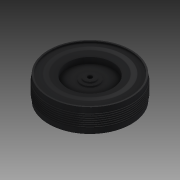
# Autodesk Inventor part: wheel
Saved by Autodesk Inventor 2016 (Build 200138000, 138)
## iProperties
Created: 2014-07-17
Part Number: wheel
Material: Rubber
Document SubType Name: Modeling
Designer: Sebastian
Density: 0.93 g/cm^3
Appearance: Rubber - Black - Version 1.1
Mass: 14.4861 g
Surface Area: 122.357 cm^2
Volume: 15.5764 cm^3
Author: Sebastian
Autodesk Inventor part; units mm, degrees
ref_plane "YZ Plane" through (0, 0, 0) normal (1, 0, 0) x (0, 1, 0)
ref_plane "XZ Plane" through (0, 0, 0) normal (0, 1, 0) x (-1, 0, 0)
ref_plane "XY Plane" through (0, 0, 0) normal (0, 0, 1) x (1, 0, 0)
sketch "Sketch1" plane through (0, 0, 0) normal (0, 1, 0) x (-1, 0, 0)
  line L0 (0, -15.5) -> (3, -15.5)
  line L1 (3, -15.5) -> (3, -3)
  line L2 (3, -3) -> (10, -3)
  line L3 (10, -3) -> (10, -8)
  line L4 (10, -8) -> (23, -8)
  line L5 (23, -8) -> (23, -19)
  line L6 (23, -19) -> (26, -19)
  line L7 (12.5, -1) -> (12.5, -5)
  line L8 (26, -19) -> (26, -5)
  line L9 (27.5, -32.1493) -> (27.5, 12.13)
  line L10 (26, -5) -> (26, -2)
  line L11 (26, -2) -> (23.5, -2)
  line L12 (23.5, -2) -> (23.5, -3)
  line L13 (23.5, -3) -> (21.5, -3)
  line L14 (21.5, -3) -> (21.5, -4)
  arc A0 (21.5, -4) -> (12.5, -5) centre (20.6098, -36.988) ccw
  line L15 (0, -15.5) -> (0, -11.75)
  line L16 (0, 0) -> (0, -3.75)
  line L17 (0, -11.75) -> (-0.5, -11.75)
  line L18 (-0.5, -11.75) -> (-0.5, -11.25)
  line L19 (-0.5, -11.25) -> (0, -11.25)
  line L20 (0, -11.25) -> (0, -10.5)
  line L21 (0, -10.5) -> (-0.5, -10.5)
  line L22 (-0.5, -10.5) -> (-0.5, -10)
  line L23 (-0.5, -10) -> (0, -10)
  line L24 (0, -10) -> (0, -9.25)
  line L25 (0, -9.25) -> (-0.5, -9.25)
  line L26 (-0.5, -9.25) -> (-0.5, -8.75)
  line L27 (-0.5, -8.75) -> (0, -8.75)
  line L28 (0, -8.75) -> (0, -8)
  line L29 (0, -8) -> (-0.5, -8)
  line L30 (-0.5, -8) -> (-0.5, -7.5)
  line L31 (-0.5, -7.5) -> (0, -7.5)
  line L32 (0, -7.5) -> (0, -6.75)
  line L33 (0, -6.75) -> (-0.5, -6.75)
  line L34 (-0.5, -6.75) -> (-0.5, -6.25)
  line L35 (-0.5, -6.25) -> (0, -6.25)
  line L36 (0, -6.25) -> (0, -5.5)
  line L37 (0, -5.5) -> (-0.5, -5.5)
  line L38 (-0.5, -5.5) -> (-0.5, -5)
  line L39 (-0.5, -5) -> (0, -5)
  line L40 (0, -5) -> (0, -4.25)
  line L41 (0, -4.25) -> (-0.5, -4.25)
  line L42 (-0.5, -4.25) -> (-0.5, -3.75)
  line L43 (-0.5, -3.75) -> (0, -3.75)
  line L44 (0, 0) -> (1, 0)
  line L45 (1, 0) -> (1, -1)
  arc A1 (12.5, -1) -> (1, -1) centre (6.75, -17.0302) ccw
  dimension "d0" = 15.5
  dimension "d1" = 3
  dimension "d2" = 12.5
  dimension "d3" = 7
  dimension "d4" = 5
  dimension "d5" = 13
  dimension "d6" = 11
  dimension "d8" = 3
  dimension "d10" = 4
  dimension "d11" = 13.5
  dimension "d12" = 26
  dimension "d16" = 3
  dimension "d17" = 2.5
  dimension "d18" = 1
  dimension "d19" = 2
  dimension "d20" = 1
  dimension "d21" = 33
  dimension "d22" = 3.75
  dimension "d23" = 3.75
  dimension "d24" = 0.5
  dimension "d25" = 0.5
  dimension "d26" = 0.75
  dimension "d27" = 0.5
  dimension "d28" = 0.75
  dimension "d29" = 0.5
  dimension "d30" = 0.75
  dimension "d31" = 0.5
  dimension "d32" = 0.75
  dimension "d33" = 0.5
  dimension "d34" = 0.75
  dimension "d35" = 0.75
  dimension "d36" = 1
  dimension "d37" = 1
  dimension "d38" = 12.5
  constraints: 92 end point, 25 perpendicular, 22 point on line, 4 point on circle, 3 horizontal, 3 vertical, 2 centre point
  measures "d0" distance of L16.start L0.start
  measures "d1" distance of L0.start L0.end
  measures "d2" distance of L0.end L1.end
  measures "d3" distance of L1.end L2.end
  measures "d4" distance of L2.end L3.end
  measures "d5" distance of L3.end L4.end
  measures "d6" distance of L4.end L5.end
  measures "d8" distance of L5.end L6.end
  measures "d10" distance of L7.start L7.end
  measures "d11" distance of L7.end L8.end
  measures "d12" horizontal distance of L0.start L6.end
  measures "d16" distance of L8.end L10.end
  measures "d17" distance of L10.end L11.end
  measures "d18" distance of L11.end L12.end
  measures "d19" distance of L12.end L13.end
  measures "d20" distance of L13.end L14.end
  measures "d21" radius of A0
  measures "d22" distance of L0.start L15.end
  measures "d23" distance of L16.start L16.end
  measures "d24" distance of L15.end L17.end
  measures "d25" distance of L17.end L18.end
  measures "d26" distance of L19.end L20.end
  measures "d27" distance of L21.end L22.end
  measures "d28" distance of L23.end L24.end
  measures "d29" distance of L25.end L26.end
  measures "d30" distance of L27.end L28.end
  measures "d31" distance of L29.end L30.end
  measures "d32" distance of L31.end L32.end
  measures "d33" distance of L33.end L34.end
  measures "d34" distance of L35.end L36.end
  measures "d35" distance of L39.end L40.end
  measures "d36" distance of L16.start L44.end
  measures "d37" distance of L44.end L45.end
  measures "d38" distance from line of L16 L7.start
revolve "Revolution1" add sketch "Sketch1" angle 360 about axis through (-27.5, 0, -32.1493) along (0, 0, 1)
body "Solid1"
